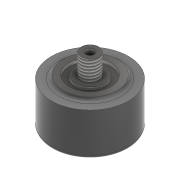
# Autodesk Inventor part: Sonar
Saved by Autodesk Inventor 2022.3 (Build 263350000, 350)
## iProperties
Created: 2023-07-17
Part Number: Sonar
Material: Genérico
Document SubType Name: Modeling
Designer: Usuario
Density: 1 g/cm^3
Appearance: Valor por defecto
Author: Usuario
Autodesk Inventor part; units mm, degrees
ref_plane "YZ Plane" through (0, 0, 0) normal (1, 0, 0) x (0, 1, 0)
ref_plane "XZ Plane" through (0, 0, 0) normal (0, 1, 0) x (-1, 0, 0)
ref_plane "XY Plane" through (0, 0, 0) normal (0, 0, 1) x (1, 0, 0)
sketch "Boceto1" plane through (0, 0, 0) normal (0, 1, 0) x (-1, 0, 0)
  circle A0 centre (0, 0) radius 20.925
  dimension "d0" = 41.85
  constraints: 1 centre point, 1 coincident
  measures "d0" diameter of A0
extrude "Extrusión1" add sketch "Boceto1" along normal blind 23.25
fillet "Empalme1" radius 2 1 edges at (20.925, 0, 0)
sketch "Boceto2" plane through (0, 23.25, 0) normal (0, 1, 0) x (1, 0, 0)
  circle A0 centre (0, 0) radius 14.75
  dimension "d4" = 29.5
  constraints: 1 centre point, 1 coincident
  measures "d4" diameter of A0
extrude "Extrusión2" add sketch "Boceto2" along normal blind 1.7
sketch "Boceto3" plane through (0, 24.95, 0) normal (0, 1, 0) x (1, 0, 0)
  circle A0 centre (0, 0) radius 11.25
  circle A1 centre (0, 0) radius 18.925 projected
  circle A2 centre (0, 0) radius 8
  dimension "d7" = 22.5
  dimension "d8" = 16
  constraints: 2 centre point, 2 coincident
  measures "d7" diameter of A0
  measures "d8" diameter of A2
extrude "Extrusión3" cut sketch "Boceto3" against normal blind 1.7 contours A0
sketch "Boceto4" plane through (0, 24.95, 0) normal (0, 1, 0) x (1, 0, 0)
  circle A0 centre (0, 0) radius 4.8
  circle A1 centre (0, 0) radius 2.35
  dimension "d11" = 9.6
  dimension "d12" = 4.7
  constraints: 2 centre point, 2 coincident
  measures "d11" diameter of A0
  measures "d12" diameter of A1
extrude "Extrusión4" add sketch "Boceto4" along normal blind 10.8
thread "Rosca1" size "M10x1.5" class "6g" standard "ANSI Metric M Profile" full length
fillet "Empalme2" radius 2 1 edges at (-14.75, 23.25, 0)
sketch "Boceto5" plane through (0, 0, 0) normal (0, -1, 0) x (1, 0, 0)
  line L0 (0.4152, 1.1019) -> (0.4152, 7.3162)
  line L1 (0.4152, 7.3162) -> (8.294, 7.3162)
  line L2 (2.1139, 1.8115) -> (2.1139, 5.6175)
  line L3 (2.1139, 5.6175) -> (8.1607, 5.6175)
  line L4 (0.4152, -3.1987) -> (0.4152, -6.7036)
  line L5 (0.4152, -6.7036) -> (2.1139, -6.7036)
  line L6 (2.1139, -6.7036) -> (2.1139, -3.0051)
  line L7 (12.8438, -6.7036) -> (12.8438, -4.9512)
  line L8 (-13.1746, 1.8115) -> (-13.1746, 0)
  arc A0 (7.7614, 0.9057) -> (8.1607, 5.6175) centre (8.1607, 3.2447) ccw
  arc A1 (8.7354, -0.6872) -> (8.294, 7.3162) centre (8.294, 3.3023) ccw
  arc A2 (0.4152, -3.1987) -> (2.1139, -3.0051) centre (1.0212, -0.9655) ccw
  arc A3 (0.4152, 1.1019) -> (2.1139, 1.8115) centre (0.7502, 2.6881) ccw
  line L9 (-13.1746, 1.8115) -> (8.294, 1.8115)
  line L10 (-8.7357, -2.0357) -> (8.4934, -2.0357)
  line L11 (-8.7357, -2.0357) -> (-13.1746, -2.0357)
  line L12 (-8.7357, -0.3398) -> (-8.7357, 1.8115)
  line L13 (0.7502, -0.3398) -> (0.7502, 1.8115)
  line L14 (5.3136, 0.142) -> (5.3136, -2.0357)
  line L15 (-3.9948, 0.142) -> (-3.9948, -2.0357)
  spline S0 degree 4 poles (-13.1746, 1.8115) (-12.7802, 1.8321) (-11.9646, 1.7566) (-11.1, 1.2176) (-10.4093, 0.5268) (-9.8572, 0.0853) (-9.3495, -0.2724) (-8.7296, -0.3826) (-8.0344, -0.2865) (-7.4628, 0.0548) (-6.8905, 0.646) (-6.1068, 1.2691) (-5.2659, 1.732) (-3.9289, 1.8643) (-2.7016, 1.7553) (-1.5553, 1.0337) (-0.8999, 0.3116) (-0.0347, -0.3302) (0.7543, -0.3828) (1.492, -0.2349) (2.3537, 0.4063) (2.8801, 1.0382) (4.2869, 1.9521) (6.2548, 1.8977) (6.872, 1.5765) (7.7614, 0.9057) knots 0 0 0 0 0 0.092739 0.12964 0.164653 0.198114 0.231161 0.263961 0.298023 0.3343 0.37251 0.414214 0.458565 0.504488 0.550766 0.595424 0.636944 0.675479 0.713523 0.751068 0.7908 0.834395 0.879268 1 1 1 1 1
  spline S1 degree 4 poles (8.7354, -0.6872) (8.9575, -1.0755) (9.5814, -2.2749) (9.868, -3.1772) (10.9462, -4.5791) (11.6643, -5.1495) (12.4847, -5.0467) (12.8438, -4.9512) knots 0 0 0 0 0 0.384708 0.534629 0.675411 1 1 1 1 1
  spline S2 degree 4 poles (-13.1746, 0) (-12.9301, 0.1461) (-11.8814, -0.1995) (-11.4975, -1.1565) (-10.0916, -1.7102) (-9.8971, -1.8746) (-8.6209, -2.1205) (-7.6745, -1.9587) (-7.0601, -1.7189) (-6.0861, -1.1842) (-5.7402, -0.6866) (-5.2056, -0.3175) (-4.6197, 0.0788) (-3.978, 0.1711) (-3.3144, 0.1346) (-2.6377, -0.3661) (-2.128, -0.9666) (-1.4055, -1.3493) (-0.7674, -1.9187) (0.8562, -2.0873) (1.8128, -2.018) (2.9082, -1.3295) (3.6709, -0.7743) (3.9605, -0.234) (5.3736, 0.31) (6.0419, -0.0065) (6.7789, -0.43) (7.2988, -1.3209) (7.5852, -1.8832) (8.134, -3.2227) (8.7384, -4.5036) (9.653, -6.1546) (10.8204, -6.472) (11.2496, -6.6926) (12.8438, -6.7036) knots 0 0 0 0 0 0.069061 0.097028 0.125152 0.15315 0.180767 0.211098 0.239513 0.266074 0.292184 0.31669 0.341267 0.366699 0.392644 0.419128 0.446624 0.476763 0.508352 0.541798 0.57509 0.605226 0.635799 0.664722 0.69351 0.723135 0.750513 0.779922 0.812402 0.84659 0.881589 0.914264 1 1 1 1 1
  point P0 (0, 0)
  point P1 (-12.4688, 1.7612)
  point P2 (-11.606, 1.4645)
  point P3 (-10.9024, 0.987)
  point P4 (-10.3656, 0.509)
  point P5 (-9.8363, 0.081)
  point P6 (-9.3216, -0.2242)
  point P7 (-8.0896, -0.2463)
  point P8 (-7.524, 0.0579)
  point P9 (-6.9221, 0.5861)
  point P10 (-6.1607, 1.1905)
  point P11 (-5.2762, 1.6301)
  point P12 (-3.9948, 1.8115)
  point P13 (-2.6878, 1.6166)
  point P14 (-1.5714, 0.9643)
  point P15 (-0.7812, 0.2623)
  point P16 (0.0381, -0.2455)
  point P17 (1.4517, -0.1665)
  point P18 (2.2492, 0.3712)
  point P19 (2.8875, 0.9655)
  point P20 (3.8447, 1.5449)
  point P21 (5.3136, 1.8115)
  point P22 (6.5191, 1.6378)
  point P23 (9.1994, -1.5698)
  point P24 (9.7361, -2.6934)
  point P25 (10.1895, -3.538)
  point P26 (10.7937, -4.3224)
  point P27 (11.4575, -4.8533)
  point P28 (12.1955, -5.0318)
  point P29 (-12.647, -0.031)
  point P30 (-11.7688, -0.5875)
  point P31 (-10.9544, -1.2939)
  point P32 (-10.1871, -1.6936)
  point P33 (-9.802, -1.8541)
  point P34 (-7.6969, -1.9284)
  point P35 (-6.9729, -1.6503)
  point P36 (-6.127, -1.1228)
  point P37 (-5.6772, -0.6875)
  point P38 (-5.1953, -0.3135)
  point P39 (-4.6066, 0.0183)
  point P40 (-3.3597, 0.0579)
  point P41 (-2.6889, -0.3704)
  point P42 (-2.1082, -0.9053)
  point P43 (-1.502, -1.3298)
  point P44 (-0.7526, -1.7685)
  point P45 (0.7502, -2.0357)
  point P46 (1.898, -1.8679)
  point P47 (2.9573, -1.2758)
  point P48 (3.6029, -0.752)
  point P49 (4.1024, -0.2889)
  point P50 (6.0783, -0.0448)
  point P51 (6.7266, -0.5132)
  point P52 (7.2329, -1.2236)
  point P53 (7.5547, -1.8553)
  point P54 (8.0837, -3.0699)
  point P55 (8.8017, -4.5808)
  point P56 (9.5521, -5.6864)
  point P57 (10.27, -6.2254)
  point P58 (10.9337, -6.5057)
  point P59 (7.7614, 0.9057)
  constraints: 32 end point, 8 perpendicular, 8 point on circle, 8 point on line, 5 vertical, 4 centre point, 3 horizontal, 2 tangent, 69 other
extrude "Extrusión5" cut sketch "Boceto5" against normal blind 1 contours L0 L9 L13 A3 | L0 L1 A1 S1 L7 S2 L10 L8 L9 S0 A0 L3 L2 | L13 L9 A3 | L9 S0 | L10 S2 | A2 L6 L5 L4
